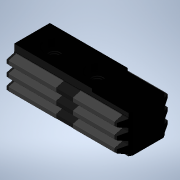
# Autodesk Inventor part: SCHUNK---Grundbacke PGN-plus-P 160-2-P
Saved by Autodesk Inventor 2021 (Build 250183000, 183)
## iProperties
Created: 2025-07-30
Part Number: SCHUNK---Grundbacke PGN-plus-P 160-2-P
Material: Generic
Catalog Web Link: www.cadenas.de
Description: Grundbacke PGN-plus P-2-finger parallel gripper
Vendor: SCHUNK
Document SubType Name: Modeling
Designer: psAdmin
Manufacturer: SCHUNK
Mass: 76.7925 g
Surface Area: 168.871 cm^2
Volume: 76.7925 cm^3
Density: 1 g/cm^3
Appearance: PSOLRGB-25-25-25
Category: PARTsolutions
Company: SCHUNK
Title: SCHUNK---Grundbacke PGN-plus-P 160-2-P
Author: Cadenas PARTsolutions
Comments: 2-finger parallel gripper
PSOL_IDENT_0: {$CADENAS_DATA/23d-libs/schunk/greifsysteme/greifmodule/greifmodule_pneumatisch/2_finger_parallelgre
PSOL_IDENT_1: ifer/2_finger_universalgreifer/pgn_plus_p/pgnplus_p_gba.prj},232 {VTYP=3D},{NB=SCHUNK---Grundbacke P
PSOL_IDENT_2: GN-plus-P 160-2-P},{LINA=SCHUNK---Grundbacke PGN-plus-P 160-2-P},{NN=Grundbacke PGN-plus P},{DATE=24
PSOL_IDENT_3: .02.2025 16:11:11},{GEOMDATE=14.08.2024 10:35:00},{VERSION=},{LINEID=320},{WBVAR=},{WBNUMERIC=}  {NB=
PSOL_IDENT_4: SCHUNK---Grundbacke PGN-plus-P 160-2-P},{LINA=SCHUNK---Grundbacke PGN-plus-P 160-2-P},{KT=DUMMY},{ID
PSOL_IDENT_5: NR=-},{TYP=PGN-plus-P 160-2-P},{L1=86.500},{P=0.200},{B1=37.860},{H1=30.0000},{B2=26.600},{H2=5.000}
PSOL_IDENT_6: ,{L1VZ=8.460},{L2VZ=8.500},{B1VZ=5.368},{B2VZ=2.539},{R1VZ=0.300},{HVZ=5.335},{H4=0.000},{L1ST=12.60
PSOL_IDENT_7: 0},{L2ST=1.500},{L3ST=5.800},{F1=23.000},{WF1=30.000},{LS1=69.540},{LS2=32.000},{SD1=15.000},{ST1=4.
PSOL_IDENT_8: 900},{G1=10.000},{GT1=17.840},{KT1=20.840},{SD2=13.600},{ST2=4.600},{L2=28.540},{H3=2.200},{TYP1=8.0
PSOL_IDENT_9: 00},{TYP2=2.000},{TYP3=1.000},{TYP4=0.000},{CNSCTN=}
NB: SCHUNK---Grundbacke PGN-plus-P 160-2-P
NN: Grundbacke PGN-plus P
NT: 2-finger parallel gripper
NBSYN: SCHUNK-$IDNR.-Grundbacke $TYP.
LINA: SCHUNK---Grundbacke PGN-plus-P 160-2-P
CATALOG: SCHUNK
IDNR: -
TYP: PGN-plus-P 160-2-P
L1: 86.5
P: 0.2
B1: 37.86
H1: 30
B2: 26.6
H2: 5
L1VZ: 8.46
L2VZ: 8.5
B1VZ: 5.368
B2VZ: 2.539
R1VZ: 0.3
HVZ: 5.335
H4: 0
L1ST: 12.6
L2ST: 1.5
L3ST: 5.8
F1: 23
WF1: 30
LS1: 69.54
LS2: 32
SD1: 15
ST1: 4.9
G1: 10
GT1: 17.84
KT1: 20.84
SD2: 13.6
ST2: 4.6
L2: 28.54
H3: 2.2
TYP1: 8
TYP2: 2
TYP3: 1
TYP4: 0
SUPPLIER: SCHUNK
ARTICLENO: SCHUNK---Grundbacke PGN-plus-P 160-2-P
BOMINFO: SCHUNK---Grundbacke PGN-plus-P 160-2-P
CREATOR: CADENAS GmbH
Autodesk Inventor part; units mm, degrees
sketch "Sketch_1" plane through (0, 0, 0) normal (0, 0, 1) x (1, 0, 0)
  line L0 (0, 30) -> (0, 0)
  line L1 (0, 0) -> (86.5, 0)
  line L2 (86.5, 0) -> (86.5, 30)
  line L3 (86.5, 30) -> (0, 30)
  constraints: 8 end point
extrude "Extrusion1" add sketch "Sketch_1" along normal mid plane 37.86
sketch "Sketch_6" plane through (0, 0, 0) normal (1, 0, 0) x (0, 1, 0)
  line L0 (25, -13.3) -> (25, -18.93)
  line L1 (25, -18.93) -> (30, -18.93)
  line L2 (30, -18.93) -> (30, -13.3)
  line L3 (30, -13.3) -> (25, -13.3)
  constraints: 8 end point
extrude "Extrusion2" cut sketch "Sketch_6" along normal blind 86.5
sketch "Sketch_7" plane through (0, 0, 0) normal (1, 0, 0) x (0, 1, 0)
  line L0 (30, 18.93) -> (25, 18.93)
  line L1 (25, 18.93) -> (25, 13.3)
  line L2 (25, 13.3) -> (30, 13.3)
  line L3 (30, 13.3) -> (30, 18.93)
  constraints: 8 end point
extrude "Extrusion3" cut sketch "Sketch_7" along normal blind 86.5
sketch "Sketch_2" plane through (0, 0, 0) normal (1, 0, 0) x (0, 1, 0)
  line L0 (25.46, -13.595) -> (24.4213, -13.595)
  arc A0 (24.4213, -13.595) -> (24.1313, -13.8181) centre (24.4213, -13.895) ccw
  line L1 (24.1313, -13.8181) -> (22.8352, -18.7069)
  arc A1 (22.5452, -18.93) -> (22.8352, -18.7069) centre (22.5452, -18.63) ccw
  line L2 (22.5452, -18.93) -> (19.8748, -18.93)
  arc A2 (19.5848, -18.7069) -> (19.8748, -18.93) centre (19.8748, -18.63) ccw
  line L3 (19.5848, -18.7069) -> (18.2887, -13.8181)
  arc A3 (18.2887, -13.8181) -> (17.9987, -13.595) centre (17.9987, -13.895) ccw
  line L4 (17.9987, -13.595) -> (15.9213, -13.595)
  arc A4 (15.9213, -13.595) -> (15.6313, -13.8181) centre (15.9213, -13.895) ccw
  line L5 (15.6313, -13.8181) -> (14.3352, -18.7069)
  arc A5 (14.0452, -18.93) -> (14.3352, -18.7069) centre (14.0452, -18.63) ccw
  line L6 (14.0452, -18.93) -> (11.3748, -18.93)
  arc A6 (11.0848, -18.7069) -> (11.3748, -18.93) centre (11.3748, -18.63) ccw
  line L7 (11.0848, -18.7069) -> (9.7887, -13.8181)
  arc A7 (9.7887, -13.8181) -> (9.4987, -13.595) centre (9.4987, -13.895) ccw
  line L8 (9.4987, -13.595) -> (7.4213, -13.595)
  arc A8 (7.4213, -13.595) -> (7.1313, -13.8181) centre (7.4213, -13.895) ccw
  line L9 (7.1313, -13.8181) -> (5.8352, -18.7069)
  arc A9 (5.5452, -18.93) -> (5.8352, -18.7069) centre (5.5452, -18.63) ccw
  line L10 (5.5452, -18.93) -> (2.9148, -18.93)
  arc A10 (2.6248, -18.7069) -> (2.9148, -18.93) centre (2.9148, -18.63) ccw
  line L11 (2.6248, -18.7069) -> (1.3287, -13.8181)
  arc A11 (1.3287, -13.8181) -> (1.0387, -13.595) centre (1.0387, -13.895) ccw
  line L12 (1.0387, -13.595) -> (0, -13.595)
  line L13 (0, -13.595) -> (0, -19.93)
  line L14 (0, -19.93) -> (25.46, -19.93)
  line L15 (25.46, -19.93) -> (25.46, -13.595)
  constraints: 32 end point, 24 point on circle, 12 centre point
extrude "Extrusion4" cut sketch "Sketch_2" along normal mid plane 173
sketch "Sketch_3" plane through (0, 0, 0) normal (1, 0, 0) x (0, 1, 0)
  line L0 (25.46, 19.93) -> (0, 19.93)
  line L1 (0, 19.93) -> (0, 13.595)
  line L2 (0, 13.595) -> (1.0387, 13.595)
  arc A0 (1.0387, 13.595) -> (1.3287, 13.8181) centre (1.0387, 13.895) ccw
  line L3 (1.3287, 13.8181) -> (2.6248, 18.7069)
  arc A1 (2.9148, 18.93) -> (2.6248, 18.7069) centre (2.9148, 18.63) ccw
  line L4 (2.9148, 18.93) -> (5.5452, 18.93)
  arc A2 (5.8352, 18.7069) -> (5.5452, 18.93) centre (5.5452, 18.63) ccw
  line L5 (5.8352, 18.7069) -> (7.1313, 13.8181)
  arc A3 (7.1313, 13.8181) -> (7.4213, 13.595) centre (7.4213, 13.895) ccw
  line L6 (7.4213, 13.595) -> (9.4987, 13.595)
  arc A4 (9.4987, 13.595) -> (9.7887, 13.8181) centre (9.4987, 13.895) ccw
  line L7 (9.7887, 13.8181) -> (11.0848, 18.7069)
  arc A5 (11.3748, 18.93) -> (11.0848, 18.7069) centre (11.3748, 18.63) ccw
  line L8 (11.3748, 18.93) -> (14.0452, 18.93)
  arc A6 (14.3352, 18.7069) -> (14.0452, 18.93) centre (14.0452, 18.63) ccw
  line L9 (14.3352, 18.7069) -> (15.6313, 13.8181)
  arc A7 (15.6313, 13.8181) -> (15.9213, 13.595) centre (15.9213, 13.895) ccw
  line L10 (15.9213, 13.595) -> (17.9987, 13.595)
  arc A8 (17.9987, 13.595) -> (18.2887, 13.8181) centre (17.9987, 13.895) ccw
  line L11 (18.2887, 13.8181) -> (19.5848, 18.7069)
  arc A9 (19.8748, 18.93) -> (19.5848, 18.7069) centre (19.8748, 18.63) ccw
  line L12 (19.8748, 18.93) -> (22.5452, 18.93)
  arc A10 (22.8352, 18.7069) -> (22.5452, 18.93) centre (22.5452, 18.63) ccw
  line L13 (22.8352, 18.7069) -> (24.1313, 13.8181)
  arc A11 (24.1313, 13.8181) -> (24.4213, 13.595) centre (24.4213, 13.895) ccw
  line L14 (24.4213, 13.595) -> (25.46, 13.595)
  line L15 (25.46, 13.595) -> (25.46, 19.93)
  constraints: 32 end point, 24 point on circle, 12 centre point
extrude "Extrusion5" cut sketch "Sketch_3" along normal mid plane 173
sketch "Sketch_4" plane through (43.25, 0, 0) normal (1, 0, 0) x (0, 0, -1)
  line L0 (13.495, 25.46) -> (13.495, 24.3213)
  arc A0 (13.495, 24.3213) -> (13.7181, 24.0313) centre (13.795, 24.3213) ccw
  line L1 (13.7181, 24.0313) -> (18.6069, 22.7352)
  arc A1 (18.83, 22.4452) -> (18.6069, 22.7352) centre (18.53, 22.4452) ccw
  line L2 (18.83, 22.4452) -> (18.83, 19.9748)
  arc A2 (18.6069, 19.6848) -> (18.83, 19.9748) centre (18.53, 19.9748) ccw
  line L3 (18.6069, 19.6848) -> (13.7181, 18.3887)
  arc A3 (13.7181, 18.3887) -> (13.495, 18.0987) centre (13.795, 18.0987) ccw
  line L4 (13.495, 18.0987) -> (13.495, 15.8213)
  arc A4 (13.495, 15.8213) -> (13.7181, 15.5313) centre (13.795, 15.8213) ccw
  line L5 (13.7181, 15.5313) -> (18.6069, 14.2352)
  arc A5 (18.83, 13.9452) -> (18.6069, 14.2352) centre (18.53, 13.9452) ccw
  line L6 (18.83, 13.9452) -> (18.83, 11.4748)
  arc A6 (18.6069, 11.1848) -> (18.83, 11.4748) centre (18.53, 11.4748) ccw
  line L7 (18.6069, 11.1848) -> (13.7181, 9.8887)
  arc A7 (13.7181, 9.8887) -> (13.495, 9.5987) centre (13.795, 9.5987) ccw
  line L8 (13.495, 9.5987) -> (13.495, 7.3213)
  arc A8 (13.495, 7.3213) -> (13.7181, 7.0313) centre (13.795, 7.3213) ccw
  line L9 (13.7181, 7.0313) -> (18.6069, 5.7352)
  arc A9 (18.83, 5.4452) -> (18.6069, 5.7352) centre (18.53, 5.4452) ccw
  line L10 (18.83, 5.4452) -> (18.83, 3.0148)
  arc A10 (18.6069, 2.7248) -> (18.83, 3.0148) centre (18.53, 3.0148) ccw
  line L11 (18.6069, 2.7248) -> (13.7181, 1.4287)
  arc A11 (13.7181, 1.4287) -> (13.495, 1.1387) centre (13.795, 1.1387) ccw
  line L12 (13.495, 1.1387) -> (13.495, 0)
  line L13 (13.495, 0) -> (19.93, 0)
  line L14 (19.93, 0) -> (19.93, 25.46)
  line L15 (19.93, 25.46) -> (13.495, 25.46)
  constraints: 32 end point, 24 point on circle, 12 centre point
extrude "Extrusion6" cut sketch "Sketch_4" along normal mid plane 12.6
sketch "Sketch_5" plane through (43.25, 0, 0) normal (1, 0, 0) x (0, 0, -1)
  line L0 (-19.93, 25.46) -> (-19.93, 0)
  line L1 (-19.93, 0) -> (-13.495, 0)
  line L2 (-13.495, 0) -> (-13.495, 1.1387)
  arc A0 (-13.495, 1.1387) -> (-13.7181, 1.4287) centre (-13.795, 1.1387) ccw
  line L3 (-13.7181, 1.4287) -> (-18.6069, 2.7248)
  arc A1 (-18.83, 3.0148) -> (-18.6069, 2.7248) centre (-18.53, 3.0148) ccw
  line L4 (-18.83, 3.0148) -> (-18.83, 5.4452)
  arc A2 (-18.6069, 5.7352) -> (-18.83, 5.4452) centre (-18.53, 5.4452) ccw
  line L5 (-18.6069, 5.7352) -> (-13.7181, 7.0313)
  arc A3 (-13.7181, 7.0313) -> (-13.495, 7.3213) centre (-13.795, 7.3213) ccw
  line L6 (-13.495, 7.3213) -> (-13.495, 9.5987)
  arc A4 (-13.495, 9.5987) -> (-13.7181, 9.8887) centre (-13.795, 9.5987) ccw
  line L7 (-13.7181, 9.8887) -> (-18.6069, 11.1848)
  arc A5 (-18.83, 11.4748) -> (-18.6069, 11.1848) centre (-18.53, 11.4748) ccw
  line L8 (-18.83, 11.4748) -> (-18.83, 13.9452)
  arc A6 (-18.6069, 14.2352) -> (-18.83, 13.9452) centre (-18.53, 13.9452) ccw
  line L9 (-18.6069, 14.2352) -> (-13.7181, 15.5313)
  arc A7 (-13.7181, 15.5313) -> (-13.495, 15.8213) centre (-13.795, 15.8213) ccw
  line L10 (-13.495, 15.8213) -> (-13.495, 18.0987)
  arc A8 (-13.495, 18.0987) -> (-13.7181, 18.3887) centre (-13.795, 18.0987) ccw
  line L11 (-13.7181, 18.3887) -> (-18.6069, 19.6848)
  arc A9 (-18.83, 19.9748) -> (-18.6069, 19.6848) centre (-18.53, 19.9748) ccw
  line L12 (-18.83, 19.9748) -> (-18.83, 22.4452)
  arc A10 (-18.6069, 22.7352) -> (-18.83, 22.4452) centre (-18.53, 22.4452) ccw
  line L13 (-18.6069, 22.7352) -> (-13.7181, 24.0313)
  arc A11 (-13.7181, 24.0313) -> (-13.495, 24.3213) centre (-13.795, 24.3213) ccw
  line L14 (-13.495, 24.3213) -> (-13.495, 25.46)
  line L15 (-13.495, 25.46) -> (-19.93, 25.46)
  constraints: 32 end point, 24 point on circle, 12 centre point
extrude "Extrusion7" cut sketch "Sketch_5" along normal mid plane 12.6
sketch "Sketch_19" plane through (43.25, 0, 0) normal (1, 0, 0) x (0, 0, -1)
  line L0 (-14.3, 24.8) -> (-13.3, 24.8)
  line L1 (-13.3, 24.8) -> (-13.3, 30)
  line L2 (-13.3, 30) -> (13.3, 30)
  line L3 (13.3, 30) -> (13.3, 24.8)
  line L4 (13.3, 24.8) -> (14.3, 24.8)
  line L5 (14.3, 24.8) -> (14.3, 31)
  line L6 (14.3, 31) -> (-14.3, 31)
  line L7 (-14.3, 31) -> (-14.3, 24.8)
  constraints: 16 end point
extrude "Extrusion8" cut sketch "Sketch_19" along normal mid plane 12.6
sketch "Sketch_8" plane through (0, 0, 0) normal (1, 0, 0) x (0, 1, 0)
  line L0 (25.46, -13.495) -> (24.3213, -13.495)
  arc A0 (24.3213, -13.495) -> (24.0313, -13.7181) centre (24.3213, -13.795) ccw
  line L1 (24.0313, -13.7181) -> (22.7352, -18.6069)
  arc A1 (22.4452, -18.83) -> (22.7352, -18.6069) centre (22.4452, -18.53) ccw
  line L2 (22.4452, -18.83) -> (19.9748, -18.83)
  arc A2 (19.6848, -18.6069) -> (19.9748, -18.83) centre (19.9748, -18.53) ccw
  line L3 (19.6848, -18.6069) -> (18.3887, -13.7181)
  arc A3 (18.3887, -13.7181) -> (18.0987, -13.495) centre (18.0987, -13.795) ccw
  line L4 (18.0987, -13.495) -> (15.8213, -13.495)
  arc A4 (15.8213, -13.495) -> (15.5313, -13.7181) centre (15.8213, -13.795) ccw
  line L5 (15.5313, -13.7181) -> (14.2352, -18.6069)
  arc A5 (13.9452, -18.83) -> (14.2352, -18.6069) centre (13.9452, -18.53) ccw
  line L6 (13.9452, -18.83) -> (11.4748, -18.83)
  arc A6 (11.1848, -18.6069) -> (11.4748, -18.83) centre (11.4748, -18.53) ccw
  line L7 (11.1848, -18.6069) -> (9.8887, -13.7181)
  arc A7 (9.8887, -13.7181) -> (9.5987, -13.495) centre (9.5987, -13.795) ccw
  line L8 (9.5987, -13.495) -> (7.3213, -13.495)
  arc A8 (7.3213, -13.495) -> (7.0313, -13.7181) centre (7.3213, -13.795) ccw
  line L9 (7.0313, -13.7181) -> (5.7352, -18.6069)
  arc A9 (5.4452, -18.83) -> (5.7352, -18.6069) centre (5.4452, -18.53) ccw
  line L10 (5.4452, -18.83) -> (3.0148, -18.83)
  arc A10 (2.7248, -18.6069) -> (3.0148, -18.83) centre (3.0148, -18.53) ccw
  line L11 (2.7248, -18.6069) -> (1.4287, -13.7181)
  arc A11 (1.4287, -13.7181) -> (1.1387, -13.495) centre (1.1387, -13.795) ccw
  line L12 (1.1387, -13.495) -> (0, -13.495)
  line L13 (0, -13.495) -> (0, -19.93)
  line L14 (0, -19.93) -> (25.46, -19.93)
  line L15 (25.46, -19.93) -> (25.46, -13.495)
  constraints: 32 end point, 24 point on circle, 12 centre point
extrude "Extrusion9" cut sketch "Sketch_8" along normal blind 1.5
sketch "Sketch_9" plane through (0, 0, 0) normal (1, 0, 0) x (0, 1, 0)
  line L0 (25.46, 19.93) -> (0, 19.93)
  line L1 (0, 19.93) -> (0, 13.495)
  line L2 (0, 13.495) -> (1.1387, 13.495)
  arc A0 (1.1387, 13.495) -> (1.4287, 13.7181) centre (1.1387, 13.795) ccw
  line L3 (1.4287, 13.7181) -> (2.7248, 18.6069)
  arc A1 (3.0148, 18.83) -> (2.7248, 18.6069) centre (3.0148, 18.53) ccw
  line L4 (3.0148, 18.83) -> (5.4452, 18.83)
  arc A2 (5.7352, 18.6069) -> (5.4452, 18.83) centre (5.4452, 18.53) ccw
  line L5 (5.7352, 18.6069) -> (7.0313, 13.7181)
  arc A3 (7.0313, 13.7181) -> (7.3213, 13.495) centre (7.3213, 13.795) ccw
  line L6 (7.3213, 13.495) -> (9.5987, 13.495)
  arc A4 (9.5987, 13.495) -> (9.8887, 13.7181) centre (9.5987, 13.795) ccw
  line L7 (9.8887, 13.7181) -> (11.1848, 18.6069)
  arc A5 (11.4748, 18.83) -> (11.1848, 18.6069) centre (11.4748, 18.53) ccw
  line L8 (11.4748, 18.83) -> (13.9452, 18.83)
  arc A6 (14.2352, 18.6069) -> (13.9452, 18.83) centre (13.9452, 18.53) ccw
  line L9 (14.2352, 18.6069) -> (15.5313, 13.7181)
  arc A7 (15.5313, 13.7181) -> (15.8213, 13.495) centre (15.8213, 13.795) ccw
  line L10 (15.8213, 13.495) -> (18.0987, 13.495)
  arc A8 (18.0987, 13.495) -> (18.3887, 13.7181) centre (18.0987, 13.795) ccw
  line L11 (18.3887, 13.7181) -> (19.6848, 18.6069)
  arc A9 (19.9748, 18.83) -> (19.6848, 18.6069) centre (19.9748, 18.53) ccw
  line L12 (19.9748, 18.83) -> (22.4452, 18.83)
  arc A10 (22.7352, 18.6069) -> (22.4452, 18.83) centre (22.4452, 18.53) ccw
  line L13 (22.7352, 18.6069) -> (24.0313, 13.7181)
  arc A11 (24.0313, 13.7181) -> (24.3213, 13.495) centre (24.3213, 13.795) ccw
  line L14 (24.3213, 13.495) -> (25.46, 13.495)
  line L15 (25.46, 13.495) -> (25.46, 19.93)
  constraints: 32 end point, 24 point on circle, 12 centre point
extrude "Extrusion10" cut sketch "Sketch_9" along normal blind 1.5
sketch "Sketch_20" plane through (0, 0, 0) normal (1, 0, 0) x (0, 1, 0)
  line L0 (24.8, 14.3) -> (24.8, 13.3)
  line L1 (24.8, 13.3) -> (30, 13.3)
  line L2 (30, 13.3) -> (30, -13.3)
  line L3 (30, -13.3) -> (24.8, -13.3)
  line L4 (24.8, -13.3) -> (24.8, -14.3)
  line L5 (24.8, -14.3) -> (31, -14.3)
  line L6 (31, -14.3) -> (31, 14.3)
  line L7 (31, 14.3) -> (24.8, 14.3)
  constraints: 16 end point
extrude "Extrusion11" cut sketch "Sketch_20" along normal blind 1.5
sketch "Sketch_10" plane through (86.5, 0, 0) normal (1, 0, 0) x (0, 0, -1)
  line L0 (13.495, 25.46) -> (13.495, 24.3213)
  arc A0 (13.495, 24.3213) -> (13.7181, 24.0313) centre (13.795, 24.3213) ccw
  line L1 (13.7181, 24.0313) -> (18.6069, 22.7352)
  arc A1 (18.83, 22.4452) -> (18.6069, 22.7352) centre (18.53, 22.4452) ccw
  line L2 (18.83, 22.4452) -> (18.83, 19.9748)
  arc A2 (18.6069, 19.6848) -> (18.83, 19.9748) centre (18.53, 19.9748) ccw
  line L3 (18.6069, 19.6848) -> (13.7181, 18.3887)
  arc A3 (13.7181, 18.3887) -> (13.495, 18.0987) centre (13.795, 18.0987) ccw
  line L4 (13.495, 18.0987) -> (13.495, 15.8213)
  arc A4 (13.495, 15.8213) -> (13.7181, 15.5313) centre (13.795, 15.8213) ccw
  line L5 (13.7181, 15.5313) -> (18.6069, 14.2352)
  arc A5 (18.83, 13.9452) -> (18.6069, 14.2352) centre (18.53, 13.9452) ccw
  line L6 (18.83, 13.9452) -> (18.83, 11.4748)
  arc A6 (18.6069, 11.1848) -> (18.83, 11.4748) centre (18.53, 11.4748) ccw
  line L7 (18.6069, 11.1848) -> (13.7181, 9.8887)
  arc A7 (13.7181, 9.8887) -> (13.495, 9.5987) centre (13.795, 9.5987) ccw
  line L8 (13.495, 9.5987) -> (13.495, 7.3213)
  arc A8 (13.495, 7.3213) -> (13.7181, 7.0313) centre (13.795, 7.3213) ccw
  line L9 (13.7181, 7.0313) -> (18.6069, 5.7352)
  arc A9 (18.83, 5.4452) -> (18.6069, 5.7352) centre (18.53, 5.4452) ccw
  line L10 (18.83, 5.4452) -> (18.83, 3.0148)
  arc A10 (18.6069, 2.7248) -> (18.83, 3.0148) centre (18.53, 3.0148) ccw
  line L11 (18.6069, 2.7248) -> (13.7181, 1.4287)
  arc A11 (13.7181, 1.4287) -> (13.495, 1.1387) centre (13.795, 1.1387) ccw
  line L12 (13.495, 1.1387) -> (13.495, 0)
  line L13 (13.495, 0) -> (19.93, 0)
  line L14 (19.93, 0) -> (19.93, 25.46)
  line L15 (19.93, 25.46) -> (13.495, 25.46)
  constraints: 32 end point, 24 point on circle, 12 centre point
extrude "Extrusion12" cut sketch "Sketch_10" against normal blind 5.8
sketch "Sketch_11" plane through (86.5, 0, 0) normal (1, 0, 0) x (0, 0, -1)
  line L0 (-19.93, 25.46) -> (-19.93, 0)
  line L1 (-19.93, 0) -> (-13.495, 0)
  line L2 (-13.495, 0) -> (-13.495, 1.1387)
  arc A0 (-13.495, 1.1387) -> (-13.7181, 1.4287) centre (-13.795, 1.1387) ccw
  line L3 (-13.7181, 1.4287) -> (-18.6069, 2.7248)
  arc A1 (-18.83, 3.0148) -> (-18.6069, 2.7248) centre (-18.53, 3.0148) ccw
  line L4 (-18.83, 3.0148) -> (-18.83, 5.4452)
  arc A2 (-18.6069, 5.7352) -> (-18.83, 5.4452) centre (-18.53, 5.4452) ccw
  line L5 (-18.6069, 5.7352) -> (-13.7181, 7.0313)
  arc A3 (-13.7181, 7.0313) -> (-13.495, 7.3213) centre (-13.795, 7.3213) ccw
  line L6 (-13.495, 7.3213) -> (-13.495, 9.5987)
  arc A4 (-13.495, 9.5987) -> (-13.7181, 9.8887) centre (-13.795, 9.5987) ccw
  line L7 (-13.7181, 9.8887) -> (-18.6069, 11.1848)
  arc A5 (-18.83, 11.4748) -> (-18.6069, 11.1848) centre (-18.53, 11.4748) ccw
  line L8 (-18.83, 11.4748) -> (-18.83, 13.9452)
  arc A6 (-18.6069, 14.2352) -> (-18.83, 13.9452) centre (-18.53, 13.9452) ccw
  line L9 (-18.6069, 14.2352) -> (-13.7181, 15.5313)
  arc A7 (-13.7181, 15.5313) -> (-13.495, 15.8213) centre (-13.795, 15.8213) ccw
  line L10 (-13.495, 15.8213) -> (-13.495, 18.0987)
  arc A8 (-13.495, 18.0987) -> (-13.7181, 18.3887) centre (-13.795, 18.0987) ccw
  line L11 (-13.7181, 18.3887) -> (-18.6069, 19.6848)
  arc A9 (-18.83, 19.9748) -> (-18.6069, 19.6848) centre (-18.53, 19.9748) ccw
  line L12 (-18.83, 19.9748) -> (-18.83, 22.4452)
  arc A10 (-18.6069, 22.7352) -> (-18.83, 22.4452) centre (-18.53, 22.4452) ccw
  line L13 (-18.6069, 22.7352) -> (-13.7181, 24.0313)
  arc A11 (-13.7181, 24.0313) -> (-13.495, 24.3213) centre (-13.795, 24.3213) ccw
  line L14 (-13.495, 24.3213) -> (-13.495, 25.46)
  line L15 (-13.495, 25.46) -> (-19.93, 25.46)
  constraints: 32 end point, 24 point on circle, 12 centre point
extrude "Extrusion13" cut sketch "Sketch_11" against normal blind 5.8
sketch "Sketch_12" plane through (0, 0, 0) normal (0, 1, 0) x (-1, 0, 0)
  line L0 (-82.2103, 18.93) -> (-87.5, 18.93)
  line L1 (-87.5, 18.93) -> (-87.5, -18.93)
  line L2 (-87.5, -18.93) -> (-82.2103, -18.93)
  line L3 (-82.2103, -18.93) -> (-86.5, -11.5)
  line L4 (-86.5, -11.5) -> (-86.5, 11.5)
  line L5 (-86.5, 11.5) -> (-82.2103, 18.93)
  constraints: 12 end point
extrude "Extrusion14" cut sketch "Sketch_12" along normal blind 30
sketch "Sketch_13" plane through (0, 0, 0) normal (0, 0, 1) x (1, 0, 0)
  line L0 (16.96, 5.1111) -> (16.96, 30)
  line L1 (16.96, 30) -> (24.8136, 30)
  line L2 (24.8136, 30) -> (24.46, 29.6464)
  line L3 (24.46, 29.6464) -> (24.46, 25.4)
  line L4 (24.46, 25.4) -> (23.76, 25.4)
  line L5 (23.76, 25.4) -> (23.76, 25.1)
  line L6 (23.76, 25.1) -> (21.148, 24.1493)
  line L7 (21.148, 24.1493) -> (21.148, 8.5025)
  line L8 (21.148, 8.5025) -> (16.96, 5.1111)
  line L9 (16.96, 5.1111) -> (16.96, 30)
  constraints: 20 end point
revolve "Revolution1" cut sketch "Sketch_13" angle 360 about axis through (16.96, 5.1111, 0) along (0, -1, 0)
thread "Thread1" size "M10x1.5" class "6H" standard "ISO Metric profile" length 12.6445
pattern_linear "Rectangular Pattern1" count 2 spacing 32 along (1, 0, 0) of "Revolution1"
sketch "Sketch_15" plane through (0, 0, 0) normal (0, 0, 1) x (1, 0, 0)
  line L0 (57.96, 30) -> (57.96, 27.8)
  line L1 (57.96, 27.8) -> (86.5, 27.8)
  line L2 (86.5, 27.8) -> (86.5, 30)
  line L3 (86.5, 30) -> (57.96, 30)
  constraints: 8 end point
extrude "Extrusion15" cut sketch "Sketch_15" along normal mid plane 37.86
ref_plane "IP_FIN_XY" through (48.96, 30, 0) normal (0, 1, 0) x (1, 0, 0)
ref_plane "IP_FIN_YZ" through (48.96, 30, 0) normal (1, 0, 0) x (0, 0, -1)
ref_plane "IP_FIN_ZX" through (48.96, 30, 0) normal (0, 0, -1) x (0, 1, 0)
ref_plane "gba_XY" through (48.96, 30, 0) normal (1, 0, 0) x (0, 0, -1)
ref_plane "gba_YZ" through (48.96, 30, 0) normal (0, 0, -1) x (0, 1, 0)
ref_plane "gba_ZX" through (48.96, 30, 0) normal (0, 1, 0) x (1, 0, 0)
ref_plane "zhu1_XY" through (16.96, 25.1, 0) normal (0, 1, 0) x (1, 0, 0)
ref_plane "zhu1_YZ" through (16.96, 25.1, 0) normal (1, 0, 0) x (0, 0, -1)
ref_plane "zhu1_ZX" through (16.96, 25.1, 0) normal (0, 0, -1) x (0, 1, 0)
ref_plane "zhu2_XY" through (48.96, 25.1, 0) normal (0, 1, 0) x (1, 0, 0)
ref_plane "zhu2_YZ" through (48.96, 25.1, 0) normal (1, 0, 0) x (0, 0, -1)
ref_plane "zhu2_ZX" through (48.96, 25.1, 0) normal (0, 0, -1) x (0, 1, 0)
body "Solid1"
